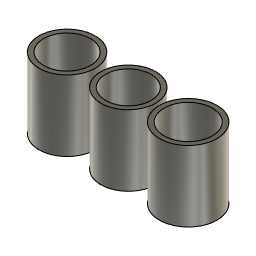
Final Project Chalk Holder v1 (Autodesk Fusion 360 design; units mm, degrees)
Autodesk Fusion 360 part; units mm, degrees
sketch "Sketch1" plane through (0, 0, 0) normal (0, 0, 1) x (1, 0, 0)
  circle A0 centre (-28.379, 38.2841) radius 5.965
  circle A1 centre (-2.6569, 38.2841) radius 6.115
  circle A2 centre (-15.379, 38.2841) radius 5.815
  dimension "d1" = 11.63
  dimension "d2" = 11.93
  dimension "d3" = 12.23
  constraint horizontal A0.centre A2.centre
  constraint horizontal A1.centre A2.centre
  measures "d1" diameter of A2
  measures "d2" diameter of A0
  measures "d3" diameter of A1
extrude "Extrude1" add sketch "Sketch1" along normal blind 15 makes body 1 at (-9.5929, 37.7051, 10) makes body 2 at (-22.4436, 37.6902, 10) makes body 3 at (3.4277, 37.6752, 10)
hole "Hole1" at (-15.379, 38.2841, 15) direction (0, 0, -1) diameter 9.63 depth 14 tip angle 180 bodies 1
hole "Hole2" at (-28.379, 38.2841, 15) direction (0, 0, -1) diameter 9.93 depth 14 tip angle 180 bodies 2
hole "Hole3" at (-2.6569, 38.2841, 15) direction (0, 0, -1) diameter 10.23 depth 14 tip angle 180 bodies 3
